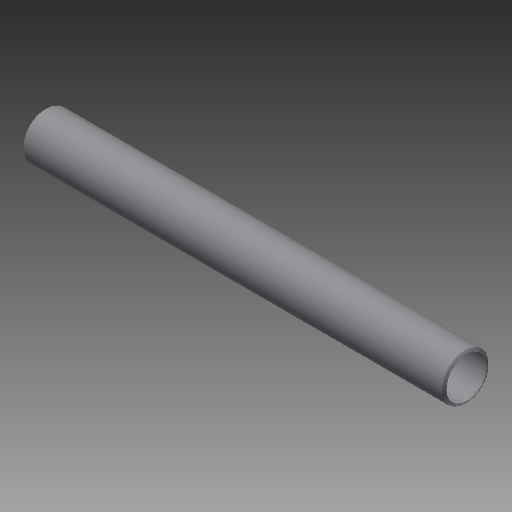
# Autodesk Inventor part: 04R-7.25550
Saved by Autodesk Inventor 2019 (Build 230136000, 136)
## iProperties
Category: PARTsolutions
Company: BIMBA
Created: 2019-01-30
Part Number: 04R-7.25550
Material: Generic
Catalog Web Link: www.cadenas.de
Description: Tube-Original Line - Standard Air Cylinders
Vendor: BIMBA
Document SubType Name: Modeling
Designer: psadmin
Manufacturer: BIMBA
Mass: 6.82129 g
Surface Area: 233.33 cm^2
Volume: 6.82129 cm^3
Density: 1 g/cm^3
Appearance: PSOLRGB-180-180-180
PSOL_IDENT_0: {$CADENAS_DATA\23d-libs\bimba\bimba\bimba_imperial\bimba_full_line\original_line_cylinders\standard_
PSOL_IDENT_1: air_cylinders\tube.prj},199 {VTYP=3D},{NB=04R-7.25550},{LINA=04R-7.25550},{NN=Tube},{DATE=21.03.2018
PSOL_IDENT_2: 14:31:21},{GEOMDATE=18.02.2011 00:00:00},{VERSION=},{LINEID=40},{WBVAR=MNT,ACTING,NR,L,FOURHOLES,SR
PSOL_IDENT_3: },{WBNUMERIC=L,FOURHOLES}  {NB=04R-7.25550},{LINA=04R-7.25550},{KT=DUMMY},{PN=04R-7.25550},{BORE=0.7
PSOL_IDENT_4: 5000000},{BOREPN=04},{MNT=},{MNTALG='' , 'Front Nose' , 'BF' , 'Front Block' , 'BFT' , 'Front Trunni
PSOL_IDENT_5: on' , 'A' , 'Adjustable Stroke'},{ACTING=R},{ACTINGALG= '' , 'Single Acting' , 'R' , 'Reverse/Double
PSOL_IDENT_6: Acting' },{NR=},{NRALG= '' , 'N/A' },{L=7.2555},{OD=0.8075},{ODN=0.8050},{ODP=0.8625},{ODB=0.8325},
PSOL_IDENT_7: {ID=0.7615},{DV=0.00000000},{LV=0.00000000},{LV1=0.00000000},{G=0.0300},{FOURHOLES=0},{AA=0.3750},{B
PSOL_IDENT_8: B=0.0940},{SR=},{SRALG= 'C' , 'Carbon Steel Rod' , 'SR' , '303 Stainless Steel Rod' , '' , '303 Stai
PSOL_IDENT_9: nless Steel Rod'}
NN: Tube
NT: Original Line - Standard Air Cylinders
NB: 04R-7.25550
NBSYN: $PN.
LINA: 04R-7.25550
BORE: 0
BOREPN: 04
MNT: Front Nose
MNTALG: '' , 'Front Nose' , 'BF' , 'Front Block' , 'BFT' , 'Front Trunnion' , 'A' , 'Adjustable Stroke'
ACTING: Reverse/Double Acting
NR: N/A
L: 7.2555
ODN: 0.805
ODP: 0.8625
ODB: 0.8325
ID: 0.7615
DV: 0
LV: 0
LV1: 0
G: 0.03
FOURHOLES: 0
AA: 0.375
BB: 0.094
SR: 303 Stainless Steel Rod
SUPPLIER: BIMBA
ARTICLENO: 04R-7.25550
BOMINFO: 04R-7.25550
CREATOR: CADENAS GmbH
Title: 04R-7.25550
Author: Cadenas PARTsolutions
Comments: Original Line - Standard Air Cylinders
Autodesk Inventor part; units mm, degrees
sketch "Sketch_1" plane through (0, 0, 0) normal (0, 0, 1) x (1, 0, 0)
  line L0 (184.2897, 0) -> (0, 0)
  arc A0 (-0.6395, 9.3472) -> (-0.6395, 9.1676) centre (-0.5497, 9.2574) ccw
  line L1 (-0.6395, 9.1676) -> (-0.381, 8.9091)
  line L2 (-0.381, 8.9091) -> (0, 8.9091)
  line L3 (0, 8.9091) -> (0.762, 9.671)
  line L4 (0.762, 9.671) -> (183.5277, 9.671)
  line L5 (183.5277, 9.671) -> (184.2897, 8.9091)
  line L6 (184.2897, 8.9091) -> (184.6707, 8.9091)
  line L7 (184.6707, 8.9091) -> (184.9292, 9.1676)
  arc A1 (184.9292, 9.1676) -> (184.9292, 9.3472) centre (184.8394, 9.2574) ccw
  line L8 (184.9292, 9.3472) -> (184.2443, 10.0321)
  arc A2 (184.2443, 10.0321) -> (183.7055, 10.2553) centre (183.7055, 9.4933) ccw
  line L9 (183.7055, 10.2553) -> (0.5842, 10.2553)
  arc A3 (0.5842, 10.2553) -> (0.0454, 10.0321) centre (0.5842, 9.4933) ccw
  line L10 (0.0454, 10.0321) -> (-0.6395, 9.3472)
  constraints: 22 end point, 8 point on circle, 4 centre point
revolve "Revolution1" add sketch "Sketch_1" angle 360 about axis through (184.2897, 0, 0) along (1, 0, 0)
ref_plane "cp1_XY" through (92.1449, 10.2553, 0) normal (1, 0, 0) x (0, 0, -1)
ref_plane "cp1_YZ" through (92.1449, 10.2553, 0) normal (0, 0, -1) x (0, 1, 0)
ref_plane "cp1_ZX" through (92.1449, 10.2553, 0) normal (0, 1, 0) x (1, 0, 0)
ref_plane "cp2_XY" through (92.1449, 0, -10.2553) normal (1, 0, 0) x (0, 0, -1)
ref_plane "cp2_YZ" through (92.1449, 0, -10.2553) normal (0, 0, -1) x (0, 1, 0)
ref_plane "cp2_ZX" through (92.1449, 0, -10.2553) normal (0, 1, 0) x (1, 0, 0)
ref_plane "cp3_XY" through (92.1449, -10.2553, 0) normal (1, 0, 0) x (0, 0, -1)
ref_plane "cp3_YZ" through (92.1449, -10.2553, 0) normal (0, 0, -1) x (0, 1, 0)
ref_plane "cp3_ZX" through (92.1449, -10.2553, 0) normal (0, 1, 0) x (1, 0, 0)
ref_plane "cp4_XY" through (92.1449, 0, 10.2553) normal (1, 0, 0) x (0, 0, -1)
ref_plane "cp4_YZ" through (92.1449, 0, 10.2553) normal (0, 0, -1) x (0, 1, 0)
ref_plane "cp4_ZX" through (92.1449, 0, 10.2553) normal (0, 1, 0) x (1, 0, 0)
ref_plane "tube_front_XY" through (0, 0, 0) normal (1, 0, 0) x (0, 0, -1)
ref_plane "tube_front_YZ" through (0, 0, 0) normal (0, 0, -1) x (0, 1, 0)
ref_plane "tube_front_ZX" through (0, 0, 0) normal (0, 1, 0) x (1, 0, 0)
ref_plane "tube_rear_XY" through (184.2897, 0, 0) normal (1, 0, 0) x (0, 0, -1)
ref_plane "tube_rear_YZ" through (184.2897, 0, 0) normal (0, 0, -1) x (0, 1, 0)
ref_plane "tube_rear_ZX" through (184.2897, 0, 0) normal (0, 1, 0) x (1, 0, 0)
body "Solid1"
